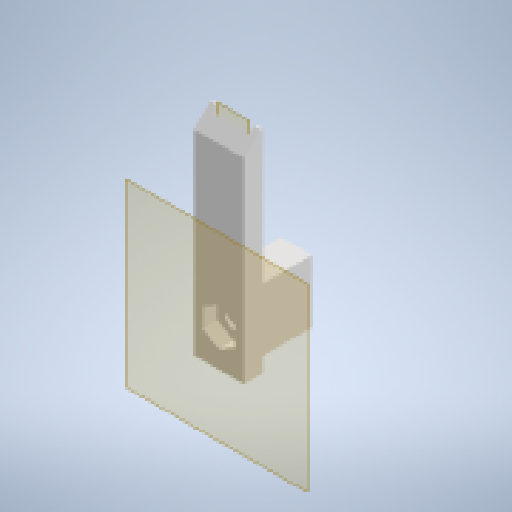
# Autodesk Inventor part: surgical_holder_side2
Saved by Autodesk Inventor 2023.3 (Build 273359000, 359)
## iProperties
Created: 2023-01-31
Part Number: surgical_holder_side2
Material: Generic
Document SubType Name: Modeling
Designer: mmelin
Density: 1 g/cm^3
Appearance: Default
Author: mmelin
Autodesk Inventor part; units mm, degrees
ref_plane "YZ Plane" through (0, 0, 0) normal (1, 0, 0) x (0, 1, 0)
ref_plane "XZ Plane" through (0, 0, 0) normal (0, 1, 0) x (-1, 0, 0)
ref_plane "XY Plane" through (0, 0, 0) normal (0, 0, 1) x (1, 0, 0)
ref_plane "Work Plane3" through (0, -0.0002, 0) normal (0, 0, 1) x (1, 0, 0)
sketch "Sketch8" plane through (0, -0.0002, 0) normal (0, 0, 1) x (1, 0, 0)
  line L0 (-0.007, 0.0002) -> (-0.007, -15.3498) projected
  line L1 (-0.007, 0.0002) -> (-4.107, 0.0002) projected
  line L2 (-4.107, 0.0002) -> (-4.107, -11.3498) projected
  line L3 (-5.107, -11.3498) -> (0.993, -11.3498)
  line L4 (0.993, -11.3498) -> (0.993, 0.0002)
  line L5 (0.993, 0.0002) -> (-5.107, 0.0002)
  line L6 (-5.107, 0.0002) -> (-5.107, -11.3498)
  line L7 (-4.107, -11.3498) -> (-1.0868, -11.3498) projected
  point P0 (-4.107, 0.0002)
  point P1 (-0.007, 0.0002)
  point P2 (-0.007, -11.3498)
  dimension "d71" = 1
  dimension "d72" = 1
  constraints: 8 end point, 2 collinear, 2 parallel, 1 horizontal, 1 perpendicular
  measures "d71" distance between parallel lines of L0 L4
  measures "d72" distance between parallel lines of L2 L6
extrude "side" add sketch "Sketch8" along normal blind 1.5
sketch "Sketch14" plane through (0, -0.0002, 0) normal (0, 0, -1) x (-1, 0, 0)
  line L0 (-0.993, 0) -> (5.107, 0) projected
  line L1 (5.107, -11.3498) -> (-0.993, -11.3498) projected
  line L2 (5.107, 0.0002) -> (4.307, 0.0002)
  line L3 (4.307, 0.0002) -> (4.307, -11.3498)
  line L4 (4.307, -11.3498) -> (5.107, -11.3498)
  line L5 (5.107, -11.3498) -> (5.107, 0.0002)
  line L6 (-0.993, -11.3498) -> (-0.193, -11.3498)
  line L7 (-0.193, -11.3498) -> (-0.193, 0.0002)
  line L8 (-0.193, 0.0002) -> (-0.993, 0.0002)
  line L9 (-0.993, 0.0002) -> (-0.993, -11.3498)
  line L10 (4.107, 0.0002) -> (4.107, -11.3498) projected
  line L11 (0.007, 0.0002) -> (0.007, -15.3498) projected
  point P0 (0, 0.0002)
  point P1 (-0.993, 0.0002)
  point P2 (-0.993, 0.0002)
  point P3 (-0.193, 0.0002)
  point P4 (4.307, 0.0002)
  dimension "d73" = 0.2
  dimension "d74" = 0.2
  constraints: 16 end point, 4 parallel, 2 horizontal, 2 perpendicular, 2 point on line, 1 other
  measures "d73" distance between parallel lines of L11 L7
  measures "d74" distance between parallel lines of L10 L3
extrude "side_tabs" add sketch "Sketch14" along normal blind 0.75 contours L0 L7 L1 L9 | L0 L5 L1 L3
sketch "Sketch15" plane through (-5.107, -11.35, 1.5) normal (0, -1, 0) x (1, 0, 0)
  line L0 (0.8, -1.5) -> (5.3, -1.5) projected
  line L1 (5.3, -1.5) -> (5.3, -2.25) projected
  line L2 (6.1, -2.25) -> (5.3, -2.25) projected
  line L3 (0, 0) -> (6.1, 0) projected
  line L4 (0.8, -2.25) -> (0, -2.25) projected
  line L5 (0.8, -1.5) -> (0.8, -2.25) projected
  line L6 (5.3, -1.5) -> (0.8, -1.5) projected
  line L7 (1, -1.5) -> (4.0182, -1.5) projected
  line L8 (0.8, -1.5) -> (0.8, -2.25) projected
  line L9 (0.8, -1.5) -> (3.8202, -1.5)
  line L10 (3.8202, -1.5) -> (3.8202, -2.008)
  line L11 (3.8202, -2.008) -> (0.8, -2.008)
  line L12 (0.8, -2.008) -> (0.8, -1.5)
  line L13 (6.1, -2.25) -> (6.1, 0) projected
  line L14 (0, 0) -> (0, -2.25) projected
  line L15 (4.0202, -1.5) -> (4.0202, -2.8009) projected
  point P0 (5.107, -1.5)
  point P1 (3.8202, -1.5)
  dimension "d99" = 0.508
  dimension "d100" = 0.2
  constraints: 8 end point, 2 parallel, 1 horizontal, 1 perpendicular
  measures "d99" distance between parallel lines of L0 L11
  measures "d100" distance between parallel lines of L15 L10
extrude "fill_gaps" add sketch "Sketch15" along normal blind 14.5
sketch "Sketch16" plane through (-5.107, -25.85, 1.5) normal (0, -1, 0) x (1, 0, 0)
  line L0 (5.3, -2.25) -> (6.1, -2.25) projected
  line L1 (5.3, -1.5) -> (5.3, -2.25) projected
  line L2 (3.8202, -1.5) -> (5.3, -1.5) projected
  line L3 (3.8202, -2.008) -> (3.8202, -1.5) projected
  line L4 (0.8, -2.008) -> (3.8202, -2.008) projected
  line L5 (0.8, -2.25) -> (0.8, -2.008) projected
  line L6 (0, -2.25) -> (0.8, -2.25) projected
  line L7 (5.3, -2.25) -> (0.8, -2.25)
  point P0 (5.107, -1.5)
  constraints: 2 end point, 1 collinear
extrude "fill_gaps_2" add sketch "Sketch16" against normal blind 9.8
chamfer "Chamfer1" distance 2 angle 45 1 edges at (-2.057, 0, 1.5)
sketch "Sketch17" plane through (0, -0.0002, -0.75) normal (0, 0, -1) x (-1, 0, 0)
  line L0 (0.007, -17.3498) -> (0.007, -25.3498) projected
  line L1 (4.107, -17.3498) -> (0.007, -17.3498) projected
  line L2 (4.107, -25.3498) -> (4.107, -17.3498) projected
  line L3 (0.007, -25.3498) -> (4.107, -25.3498) projected
  line L4 (0.182, -25.1748) -> (3.932, -25.1748)
  line L5 (3.932, -25.1748) -> (3.932, -17.5248)
  line L6 (3.932, -17.5248) -> (0.182, -17.5248)
  line L7 (0.182, -17.5248) -> (0.182, -25.1748)
  point P0 (0, 0.0002)
  dimension "d86" = 0.175
  dimension "d87" = 0.175
  dimension "d88" = 0.175
  dimension "d89" = 0.175
  constraints: 8 end point, 2 parallel, 1 horizontal, 1 perpendicular
  measures "d86" distance between parallel lines of L3 L4
  measures "d87" distance between parallel lines of L2 L5
  measures "d88" distance between parallel lines of L1 L6
  measures "d89" distance between parallel lines of L7 L0
extrude "sliding_block" add sketch "Sketch17" along normal blind 7.2 contours L7 L6 L5 L4
ref_plane "Work Plane4" through (-2.2725, -22.3901, 1.5) normal (0, 0, 1) x (1, 0, 0)
sketch "Sketch19" plane through (-2.2725, -22.3901, 1.5) normal (0, 0, 1) x (1, 0, 0)
  circle A0 centre (0.2155, 1.0401) radius 1.15 projected
  point P0 (2.2725, 22.3901)
extrude "screw_hole" cut sketch "Sketch19" against normal through all
sketch "Sketch20" plane through (0, -0.0002, 1.5) normal (0, 0, 1) x (1, 0, 0)
  line L0 (-2.057, -19.0404) -> (-0.057, -20.1951)
  line L1 (-0.057, -20.1951) -> (-0.057, -22.5045)
  line L2 (-0.057, -22.5045) -> (-2.057, -23.6592)
  line L3 (-2.057, -23.6592) -> (-4.057, -22.5045)
  line L4 (-4.057, -22.5045) -> (-4.057, -20.1951)
  line L5 (-4.057, -20.1951) -> (-2.057, -19.0404)
  circle A0 centre (-2.057, -21.3498) radius 1.15 projected
  point P0 (0, 0.0002)
  dimension "d102" = 4
  constraints: 12 end point, 1 coincident, 1 vertical, 13 other
  measures "d102" distance between parallel lines of L4 L1
extrude "nut_slot" cut sketch "Sketch20" against normal blind 1.8 contours L0 L1 L2 L3 L4 L5 | A0
equation "\"d73\" = d74"
equation "\"d86\" = d89"
equation "\"d87\" = d89"
equation "\"d88\" = d89"
body "Solid2"
